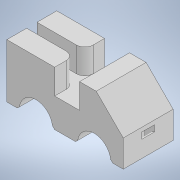
# Autodesk Inventor part: Magnet Mount Lower
Saved by Autodesk Inventor 2022 (Build 260153000, 153)
## iProperties
Created: 2022-04-23
Part Number: Magnet Mount Lower
Material: Generic
Document SubType Name: Modeling
Designer: Nick
Density: 1 g/cm^3
Appearance: Default
Author: Nick
Autodesk Inventor part; units mm, degrees
ref_plane "YZ Plane" through (0, 0, 0) normal (1, 0, 0) x (0, 1, 0)
ref_plane "XZ Plane" through (0, 0, 0) normal (0, 1, 0) x (-1, 0, 0)
ref_plane "XY Plane" through (0, 0, 0) normal (0, 0, 1) x (1, 0, 0)
sketch "Sketch1" plane through (0, 0, 0) normal (0, 0, 1) x (1, 0, 0)
  line L0 (0, 0) -> (28, 0)
  line L1 (28, 0) -> (28, 13)
  line L2 (28, 13) -> (0, 13)
  line L3 (0, 13) -> (0, 0)
  circle A0 centre (7, 0) radius 4
  circle A1 centre (21, 0) radius 4
  point P0 (3, 0)
  point P1 (11, 0)
  point P2 (17, 0)
  point P3 (25, 0)
  dimension "d0" = 28
  dimension "d1" = 13
  dimension "d2" = 8
  dimension "d3" = 8
  dimension "d4" = 14
  dimension "d5" = 7
  dimension "d6" = 7
  constraints: 8 end point, 2 centre point, 2 parallel, 2 point on line, 1 horizontal, 1 perpendicular
  measures "d0" distance of L1.end L2.end
  measures "d1" distance of L0.end L1.end
  measures "d2" diameter of A0
  measures "d3" diameter of A1
  measures "d4" distance of A1.centre A0.centre
  measures "d5" distance from line of L1 A1.centre
  measures "d6" distance from line of A0.centre L3
extrude "Extrusion1" add sketch "Sketch1" along normal blind 12 contours A1 L0 A0 L3 L2 L1
chamfer "Chamfer1" distance 6.5 angle 45 1 edges at (28, 13, 6)
sketch "Sketch2" plane through (0, 13, 12) normal (0, 1, 0) x (1, 0, 0)
  line L0 (0, 12) -> (0, 0) projected
  line L1 (0, 7.25) -> (11.5, 7.25)
  line L2 (11.5, 7.25) -> (11.5, 12)
  line L3 (21.5, 12) -> (0, 12) projected
  line L4 (17.5, 12) -> (17.5, 0)
  line L5 (11, 0) -> (17, 0) projected
  line L6 (0, 4.75) -> (11.5, 4.75)
  line L7 (11.5, 4.75) -> (11.5, 0)
  line L8 (11, 0) -> (3, 0) projected
  line L9 (11.5, 12) -> (17.5, 12)
  line L10 (25, 12) -> (17, 12) projected
  line L11 (17.5, 0) -> (11.5, 0)
  line L12 (0, 4.75) -> (0, 7.25)
  dimension "d12" = 6
  dimension "d13" = 2.5
  dimension "d14" = 11.5
  constraints: 16 end point, 6 point on line, 3 collinear, 3 perpendicular, 2 horizontal, 1 parallel, 1 vertical
  measures "d12" distance between parallel lines of L4 L2
  measures "d13" distance between parallel lines of L6 L1
  measures "d14" distance of L1.start L1.end
extrude "Extrusion2" cut sketch "Sketch2" against normal blind 6 contours L1 L2 L3 L4 L11 L5 L7 L6 L0
fillet "Fillet1" radius 2 2 edges at (11.5, 10, 4.75) (11.5, 10, 7.25)
chamfer "Chamfer2" distance 0.5 angle 45 4 edges at (3, 0, 6) (11, 0, 6) (17, 0, 6) (25, 0, 6)
ref_plane "Work Plane1" through (0, 0, 6) normal (0, 0, 1) x (1, 0, 0)
sketch "Sketch3" plane through (28, 0, 12) normal (1, 0, 0) x (0, 0, -1)
  line L0 (4.5, 5.5) -> (7.5, 5.5)
  line L1 (7.5, 5.5) -> (7.5, 4)
  line L2 (7.5, 4) -> (4.5, 4)
  line L3 (4.5, 4) -> (4.5, 5.5)
  line L4 (12, 0) -> (0, 0) projected
  line L5 (12, 0) -> (12, 6.5) projected
  line L6 (0, 6.5) -> (12, 6.5) projected
  point P0 (6, 4)
  point P1 (6, 0)
  point P2 (7.5, 4.75)
  point P3 (12, 3.25)
  dimension "d21" = 3
  dimension "d22" = 1.5
  dimension "d25" = 1
  constraints: 8 end point, 4 midpoint, 2 parallel, 1 horizontal, 1 perpendicular, 1 vertical alignment
  measures "d21" distance of L1.end L2.end
  measures "d22" distance of L0.end L1.end
  measures "d25" distance between parallel lines of L6 L0
sketch "Sketch4" plane through (0, 0, 6) normal (0, 0, 1) x (1, 0, 0)
  line L0 (28, 5.5) -> (28, 4) projected
  line L1 (26.4844, 3.2344) -> (26.4844, -0.002)
  line L2 (24.9688, 0.499) -> (25.5, 0) projected
  line L3 (24.9688, 0.499) -> (28, 0.499)
  arc A0 (28, 4.75) -> (26.4844, 3.2344) centre (28, 3.2344) ccw
  line L4 (28, 4.75) -> (27.1869, 4.75) construction
  line L5 (28, 0) -> (28, 6.5) projected
  point P0 (0, 0)
  point P1 (26.4844, 0.499)
  constraints: 6 end point, 2 horizontal, 2 midpoint, 2 point on circle, 2 point on line, 2 tangent, 1 centre point, 1 vertical
sweep "Sweep1" cut profiles "Sketch3" path "Sketch4" path curves A0 L1
ref_plane "Work Plane2" through (14, 0, 12) normal (1, 0, 0) x (0, 0, -1)
mirror "Mirror1" about plane through (14, 0, 12) normal (1, 0, 0) of "Sweep1"
equation "\"d5\" = d6"
body "Solid1"
